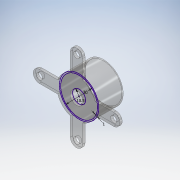
# Autodesk Inventor part: Pok Mk 3 Yaw Motor Mount
Saved by Autodesk Inventor 2018.2 (Build 222227000, 227)
## iProperties
Created: 2018-02-27
Part Number: Pok Mk 3 Yaw Motor Mount
Material: Generic
Document SubType Name: Modeling
Designer: Moochster
Density: 1 g/cm^3
Appearance: Light Gray Reflective
Author: Moochster
Autodesk Inventor part; units mm, degrees
ref_plane "YZ Plane" through (0, 0, 0) normal (1, 0, 0) x (0, 1, 0)
ref_plane "XZ Plane" through (0, 0, 0) normal (0, 1, 0) x (-1, 0, 0)
ref_plane "XY Plane" through (0, 0, 0) normal (0, 0, 1) x (1, 0, 0)
sketch "Sketch1" plane through (0, 0, 0) normal (0, 1, 0) x (-1, 0, 0)
  circle A0 centre (0, 0) radius 15
  circle A1 centre (0, 0) radius 16
  circle A2 centre (0, 0) radius 5.25
  dimension "d0" = 30
  dimension "d1" = 1
  dimension "d6" = 10.5
  constraints: 3 centre point, 3 coincident
  measures "d0" diameter of A0
  measures "d1" radial gap between concentric circles of A0 A1
  measures "d6" diameter of A2
extrude "Extrusion1" add sketch "Sketch1" along normal blind 20 contours A1
extrude "Extrusion2" add sketch "Sketch1" against normal blind 2 contours A0 | A1
sketch "Sketch3" plane through (0, -2, 0) normal (0, -1, 0) x (1, 0, 0)
  circle A0 centre (0, 0) radius 16 projected
  line L0 (15.1987, 5) -> (30.1987, 5)
  arc A1 (30.1987, -5) -> (30.1987, 5) centre (30.1987, 0) ccw
  line L1 (30.1987, -5) -> (15.1987, -5)
  circle A2 centre (30.1987, 0) radius 2.5
  dimension "d9" = 5
  dimension "d10" = 15
  dimension "d13" = 5
  constraints: 4 end point, 4 point on circle, 2 centre point, 2 tangent, 1 coincident, 1 horizontal, 1 horizontal alignment, 1 parallel
  measures "d9" distance from line of A1.centre L1
  measures "d10" distance of L1.start L1.end
  measures "d13" diameter of A2
extrude "Extrusion3" add sketch "Sketch3" against normal blind 2 contours A0 L0 A1 L1
pattern_circular "Circular Pattern1" count 4 over 360 about axis through (0, 0, 0) along (0, 1, 0) of "Extrusion3"
body "Solid1"
